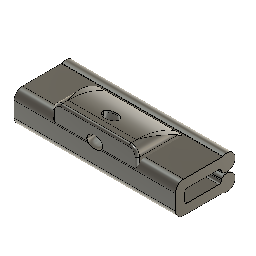
pull-string v12 (Autodesk Fusion 360 design; units mm, degrees)
Autodesk Fusion 360 part; units mm, degrees
note: some values were not read from the file. Chosen so that the rebuilt part matches the saved one: which pieces of a blend or face edit are solid.
sketch "negative" plane through (0, 0, 0) normal (1, 0, 0) x (0, 1, 0)
  line L0 (7.85, -3.3) -> (-7.85, -3.3)
  line L1 (-9.15, -2) -> (-9.15, 2)
  line L2 (-7.85, 3.3) -> (7.85, 3.3)
  line L3 (9.15, 2) -> (9.15, -2)
  line L4 (9.15, -3.3) -> (-9.15, 3.3) construction
  line L5 (-9.15, -3.3) -> (9.15, 3.3) construction
  arc A0 (-7.85, 3.3) -> (-9.15, 2) centre (-7.85, 2) ccw
  arc A1 (9.15, 2) -> (7.85, 3.3) centre (7.85, 2) ccw
  arc A2 (7.85, -3.3) -> (9.15, -2) centre (7.85, -2) ccw
  arc A3 (-9.15, -2) -> (-7.85, -3.3) centre (-7.85, -2) ccw
  line L6 (9.15, -6.3) -> (-9.15, -6.3)
  line L7 (-12.15, -3.3) -> (-12.15, 3.3)
  line L8 (-9.15, 6.3) -> (9.15, 6.3)
  line L9 (12.15, 3.3) -> (12.15, -3.3)
  line L10 (12.15, -6.3) -> (-12.15, 6.3) construction
  line L11 (-12.15, -6.3) -> (12.15, 6.3) construction
  arc A4 (12.15, 3.3) -> (9.15, 6.3) centre (9.15, 3.3) ccw
  arc A5 (9.15, -6.3) -> (12.15, -3.3) centre (9.15, -3.3) ccw
  arc A6 (-12.15, -3.3) -> (-9.15, -6.3) centre (-9.15, -3.3) ccw
  arc A7 (-9.15, 6.3) -> (-12.15, 3.3) centre (-9.15, 3.3) ccw
  circle A8 centre (11.9721, 4.3178) radius 4
  circle A9 centre (11.9721, -4.3178) radius 4
  line L12 (-9.65, -7.8) -> (9.65, -7.8)
  line L13 (13.65, -3.8) -> (13.65, 3.8)
  line L14 (9.65, 7.8) -> (-9.65, 7.8)
  line L15 (-13.65, 3.8) -> (-13.65, -3.8)
  line L16 (-13.65, -7.8) -> (13.65, 7.8) construction
  line L17 (13.65, -7.8) -> (-13.65, 7.8) construction
  arc A10 (-9.65, 7.8) -> (-13.65, 3.8) centre (-9.65, 3.8) ccw
  arc A11 (-13.65, -3.8) -> (-9.65, -7.8) centre (-9.65, -3.8) ccw
  arc A12 (9.65, -7.8) -> (13.65, -3.8) centre (9.65, -3.8) ccw
  arc A13 (13.65, 3.8) -> (9.65, 7.8) centre (9.65, 3.8) ccw
  dimension "d1" = 6.6
  dimension "d2" = 18.3
  dimension "d3" = 1.3
  dimension "d4" = 3
  dimension "d5" = 3
  dimension "d6" = 3
  dimension "d8" = 8
  dimension "d9" = 8
  dimension "d12" = 4.5
  dimension "d13" = 4.5
  dimension "d14" = 4
  constraint horizontal L0
  constraint perpendicular L0 L1
  constraint parallel L0 L2
  constraint parallel L1 L3
  constraint coincident L4 origin
  constraint coincident L5 origin
  constraint coincident L4.end L2
  constraint coincident L4.end L1
  constraint tangent L2 A0
  constraint tangent L1 A0
  constraint coincident L5.end L2
  constraint coincident L5.end L3
  constraint tangent L2 A1
  constraint tangent L3 A1
  constraint equal A0 A1
  constraint coincident L4.start L3
  constraint coincident L4.start L0
  constraint tangent L3 A2
  constraint tangent L0 A2
  constraint equal A0 A2
  constraint coincident L5.start L1
  constraint coincident L5.start L0
  constraint tangent L1 A3
  constraint tangent L0 A3
  constraint equal A0 A3
  constraint horizontal L6
  constraint perpendicular L6 L7
  constraint parallel L6 L8
  constraint parallel L7 L9
  constraint coincident L10 origin
  constraint coincident L11 origin
  constraint coincident L11.end L8
  constraint coincident L11.end L9
  constraint tangent L8 A4
  constraint tangent L9 A4
  constraint coincident L10.start L9
  constraint coincident L10.start L6
  constraint tangent L9 A5
  constraint tangent L6 A5
  constraint equal A4 A5
  constraint coincident L11.start L6
  constraint coincident L11.start L7
  constraint tangent L6 A6
  constraint tangent L7 A6
  constraint equal A4 A6
  constraint coincident L10.end L7
  constraint coincident L10.end L8
  constraint tangent L7 A7
  constraint tangent L8 A7
  constraint equal A4 A7
  constraint coincident A4 A8.centre
  constraint coincident A5 A9.centre
  constraint horizontal L12
  constraint perpendicular L12 L13
  constraint parallel L12 L14
  constraint parallel L13 L15
  constraint coincident L16 origin
  constraint coincident L17 origin
  constraint coincident L17.end L14
  constraint coincident L17.end L15
  constraint tangent L14 A10
  constraint tangent L15 A10
  constraint coincident L16.start L15
  constraint coincident L16.start L12
  constraint tangent L15 A11
  constraint tangent L12 A11
  constraint equal A10 A11
  constraint coincident L17.start L12
  constraint coincident L17.start L13
  constraint tangent L12 A12
  constraint tangent L13 A12
  constraint equal A10 A12
  constraint coincident L16.end L13
  constraint coincident L16.end L14
  constraint tangent L13 A13
  constraint tangent L14 A13
  constraint equal A10 A13
  measures "d1" distance of L0 L2
  measures "d2" distance of L1 L3
  measures "d3" radius of A0
  measures "d4" distance of L2 L8
  measures "d5" distance of L1 L7
  measures "d6" radius of A4
  measures "d8" diameter of A8
  measures "d9" diameter of A9
  measures "d12" distance of L2 L14
  measures "d13" distance of L1 L15
  measures "d14" radius of A10
extrude "Extrude2" add sketch "negative" along normal mid plane 80 contours L0 L1 L2 A0 A1 A2 A3 L6 L7 L8 A6 A7 A8 A9 | L3 A2 L6 L9 A5 A9 | L6 L7 L8 A6 A7 A8 A9 L12 L14 L15 A10 A11 A12 A13 | L6 L9 A5 A9 L13 A12 | L3 A1 L8 L9 A4 A8 | A9 L13 A12 | L8 L9 A4 A8 L13 A13 | A8 L13 A13
sketch "Sketch2" plane through (0, 0, 0) normal (0, 1, 0) x (1, 0, 0)
  line L0 (-20.9754, -4.3974) -> (21.0246, -4.3974)
  line L1 (21.0246, -4.3974) -> (21.0246, -9.3974)
  line L2 (17.0246, -13.3974) -> (-16.9754, -13.3974)
  line L3 (-20.9754, -9.3974) -> (-20.9754, -4.3974)
  line L4 (-20.9754, -4.3974) -> (21.0246, -13.3974) construction
  line L5 (21.0246, -4.3974) -> (-20.9754, -13.3974) construction
  arc A0 (17.0246, -13.3974) -> (21.0246, -9.3974) centre (17.0246, -9.3974) ccw
  arc A1 (-20.9754, -9.3974) -> (-16.9754, -13.3974) centre (-16.9754, -9.3974) ccw
  point P0 (0.0246, -8.8974)
  dimension "d17" = 42
  dimension "d18" = 9
  dimension "d19" = 4
  constraint horizontal L0
  constraint perpendicular L0 L1
  constraint parallel L0 L2
  constraint parallel L1 L3
  constraint coincident L4 P0
  constraint coincident L5 P0
  constraint coincident L4.end L1
  constraint coincident L4.end L2
  constraint tangent L1 A0
  constraint tangent L2 A0
  constraint coincident L5.end L2
  constraint coincident L5.end L3
  constraint tangent L2 A1
  constraint tangent L3 A1
  constraint equal A0 A1
  measures "d17" distance of L1 L3
  measures "d18" distance of L0 L2
  measures "d19" radius of A0
extrude "Extrude3" add sketch "Sketch2" along normal blind 9
extrude "Extrude7" add sketch "Sketch2" against normal blind 13.6
fillet "Fillet1" radius 1 5 edges at (21.0246, -13.6, 6.9139) (19.8531, -13.6, 12.2258) (0.0246, -13.6, 13.3974) (-19.8038, -13.6, 12.2258) (-20.9754, -13.6, 6.9139)
fillet "Fillet2" radius 35 5 edges at (-19.8038, 9, 12.2258) (0.0246, 9, 13.3974) (19.8531, 9, 12.2258) (21.0246, 9, 8.5987) (-20.9754, 9, 8.5987)
ref_plane "WorkPlane2" through (0, -12, 0) normal (0, 1, 0) x (0, 0, 1)
ref_plane "WorkPlane3" through (0, 0, 12) normal (0, 0, 1) x (1, 0, 0)
sketch "hole" plane through (0, 0, 12) normal (0, 0, 1) x (1, 0, 0)
  ellipse E0 centre (0, -5.5) end of major axis (4, -5.5) minor radius 2.8493
  line L0 (-4, -5.5) -> (4, -5.5)
  line L1 (0, -8.3493) -> (0, -2.6507)
  constraint coincident E0 L0.start
  constraint coincident E0 L0.end
  constraint coincident E0 L1.start
  constraint coincident E0 L1.end
  constraint horizontal L0
revolve "Revolve1" cut sketch "hole" angle 360 about axis through (-16.902, -12, 12) along (1, 0, 0)
extrude "Extrude5" cut sketch "negative" along normal mid plane 200 contours L0 L1 L2 L3 A0 A1 A2 A3 A8 A9 | L3 A2 A9 | L3 A1 A8
